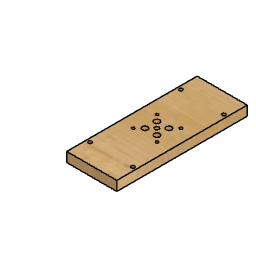
GaugePlate (Autodesk Fusion 360 design; units mm, degrees)
Autodesk Fusion 360 part; units mm, degrees
note: some values were not read from the file. Set by a fixed rule: which sketch regions a step uses.
sketch "Sketch1" plane through (-259.7942, 1290.9997, 156.4644) normal (0, 0, -1) x (0, -1, 0)
  arc A0 (507.289, -372.5213) -> (507.289, -319.0933) centre (371.7199, -345.8073) ccw
  arc A1 (507.289, -319.0933) -> (502.554, -315.2003) centre (502.554, -320.0263) ccw
  line L0 (502.554, -315.2003) -> (467.3804, -315.2003)
  arc A2 (467.3804, -315.2003) -> (465.9577, -315.4148) centre (467.3804, -320.0263) ccw
  arc A3 (452.8026, -315.6592) -> (465.9577, -315.4148) centre (458.9562, -292.7213) ccw
  arc A4 (452.8026, -315.6592) -> (450.3016, -315.6592) centre (451.5521, -320.3204) ccw
  arc A5 (437.9944, -315.6592) -> (450.3016, -315.6592) centre (444.148, -292.7213) ccw
  arc A6 (437.9944, -315.6592) -> (435.4934, -315.6592) centre (436.7439, -320.3204) ccw
  arc A7 (423.1862, -315.6592) -> (435.4934, -315.6592) centre (429.3398, -292.7213) ccw
  arc A8 (423.1862, -315.6592) -> (420.6852, -315.6592) centre (421.9357, -320.3204) ccw
  arc A9 (407.5301, -315.4148) -> (420.6852, -315.6592) centre (414.5316, -292.7213) ccw
  arc A10 (407.5301, -315.4148) -> (406.1074, -315.2003) centre (406.1074, -320.0263) ccw
  line L1 (406.1074, -315.2003) -> (370.9579, -315.2003)
  circle A11 centre (370.9579, -318.3753) radius 3.175
  line L2 (370.9579, -315.2003) -> (370.9338, -315.2003)
  arc A12 (370.9338, -315.2003) -> (366.1989, -319.0933) centre (370.9338, -320.0263) ccw
  arc A13 (366.1989, -319.0933) -> (366.1989, -372.5213) centre (501.7679, -345.8073) ccw
  arc A14 (366.1989, -372.5213) -> (370.9338, -376.4143) centre (370.9338, -371.5883) ccw
  line L3 (370.9338, -376.4143) -> (406.1074, -376.4143)
  arc A15 (406.1074, -376.4143) -> (407.5301, -376.1998) centre (406.1074, -371.5883) ccw
  arc A16 (420.6852, -375.9554) -> (407.5301, -376.1998) centre (414.5316, -398.8933) ccw
  arc A17 (420.6852, -375.9554) -> (423.1862, -375.9554) centre (421.9357, -371.2942) ccw
  arc A18 (435.4934, -375.9554) -> (423.1862, -375.9554) centre (429.3398, -398.8933) ccw
  arc A19 (435.4934, -375.9554) -> (437.9944, -375.9554) centre (436.7439, -371.2942) ccw
  arc A20 (450.3016, -375.9554) -> (437.9944, -375.9554) centre (444.148, -398.8933) ccw
  arc A21 (450.3016, -375.9554) -> (452.8026, -375.9554) centre (451.5521, -371.2942) ccw
  arc A22 (465.9577, -376.1998) -> (452.8026, -375.9554) centre (458.9562, -398.8933) ccw
  arc A23 (465.9577, -376.1998) -> (467.3804, -376.4143) centre (467.3804, -371.5883) ccw
  line L4 (467.3804, -376.4143) -> (502.5299, -376.4143)
  circle A24 centre (502.5299, -373.2393) radius 3.175
  line L5 (502.5299, -376.4143) -> (502.554, -376.4143)
  arc A25 (502.554, -376.4143) -> (507.289, -372.5213) centre (502.554, -371.5883) ccw
  circle A26 centre (500.2312, -363.2317) radius 0.8455
  circle A27 centre (472.3166, -363.2317) radius 0.8455
  circle A28 centre (379.5939, -318.8198) radius 2.159
  circle A29 centre (379.5939, -372.7948) radius 2.159
  circle A30 centre (478.3364, -363.2317) radius 2.159
  circle A31 centre (494.2114, -363.2317) radius 2.159
  circle A32 centre (493.8939, -372.7948) radius 2.159
  circle A33 centre (493.8939, -318.8198) radius 2.159
  circle A34 centre (436.7439, -345.8073) radius 6.35
  arc A35 (376.4189, -329.4243) -> (372.7359, -333.1073) centre (376.4189, -333.1073) ccw
  line L6 (376.4189, -329.4243) -> (382.7689, -329.4243)
  arc A36 (386.4519, -333.1073) -> (382.7689, -329.4243) centre (382.7689, -333.1073) ccw
  line L7 (386.4519, -333.1073) -> (386.4519, -358.5073)
  arc A37 (382.7689, -362.1903) -> (386.4519, -358.5073) centre (382.7689, -358.5073) ccw
  line L8 (382.7689, -362.1903) -> (376.4189, -362.1903)
  arc A38 (372.7359, -358.5073) -> (376.4189, -362.1903) centre (376.4189, -358.5073) ccw
  line L9 (372.7359, -358.5073) -> (372.7359, -333.1073)
  circle A39 centre (371.7439, -373.3073) radius 2.413
  circle A40 centre (501.7439, -318.3073) radius 2.413
  line L10 (518.7439, -314.3073) -> (354.7439, -314.3073)
  line L11 (354.7439, -314.3073) -> (354.7439, -377.3073)
  line L12 (354.7439, -377.3073) -> (518.7439, -377.3073)
  line L13 (518.7439, -377.3073) -> (518.7439, -314.3073)
  circle A41 centre (493.8939, -318.8198) radius 2.159
  circle A42 centre (493.8939, -372.7948) radius 2.159
  circle A43 centre (379.5939, -318.8198) radius 2.159
  circle A44 centre (379.5939, -372.7948) radius 2.159
  circle A45 centre (436.7439, -345.8073) radius 2.3876
  dimension "GaugePlateLength" = 164
  dimension "GaugePlateWidth" = 63
  dimension "d106" = 82
  dimension "d107" = 31.5
  constraint horizontal L10
  constraint vertical L11
  constraint horizontal L12
  constraint vertical L13
  constraint concentric A33 A41
  constraint concentric A32 A42
  constraint concentric A28 A43
  constraint concentric A29 A44
  measures "GaugePlateLength" distance of L10.start L10.end
  measures "GaugePlateWidth" distance of L10.start L12.end
  measures "d106" distance of A34.centre L13
  measures "d107" distance of A34.centre L10
extrude "Extrude1" add sketch "Sketch1" along normal blind 12.1 contours A0 A1 L0 A2 A3 A4 A5 A6 A7 A8 A9 A10 L1 A11 A12 A13 A14 L3 A15 A16 A17 A18 A19 A20 A21 A22 A23 L4 A24 A25 | A24 L5 | A11 L2 | A26 | A27 | A30 | A31 | A34 | A35 L6 A36 L7 A37 L8 A38 L9 | A39 | A40 | L10 L11 L12 L13
move_body "Move1" bodies 1 to x (1, 0, 0) y (0, 1, 0) z (0, 0, 1) at (0, -10, 0)
sketch "Sketch2" plane through (0, 0, 156.4644) normal (0, 0, 1) x (-1, 0, 0)
  circle A0 centre (-493.8939, -308.8198) radius 2.159
  circle A1 centre (-493.8939, -362.7948) radius 2.159
  circle A2 centre (-379.5939, -362.7948) radius 2.159
  circle A3 centre (-379.5939, -308.8198) radius 2.159
  line L0 (-518.7439, -304.3073) -> (-518.7439, -367.3073)
  line L1 (-518.7439, -367.3073) -> (-354.7439, -367.3073)
  line L2 (-354.7439, -367.3073) -> (-354.7439, -304.3073)
  line L3 (-354.7439, -304.3073) -> (-518.7439, -304.3073)
  circle A4 centre (-616.7439, -343.8073) radius 1.75
  circle A5 centre (-646.7439, -343.8073) radius 1.75
  circle A6 centre (-616.7439, -313.8073) radius 1.75
  circle A7 centre (-646.7439, -313.8073) radius 1.75
  circle A8 centre (-436.7439, -335.8073) radius 2.3876
sketch "Sketch3" plane through (0, 0, 156.4644) normal (0, 0, 1) x (-1, 0, 0)
  circle A0 centre (-59.0256, -787.1058) radius 2.159
  circle A1 centre (-113.0006, -787.1058) radius 2.159
  circle A2 centre (-113.0006, -901.4058) radius 2.159
  circle A3 centre (-59.0256, -901.4058) radius 2.159
  line L0 (-54.5131, -762.2558) -> (-117.5131, -762.2558)
  line L1 (-117.5131, -762.2558) -> (-117.5131, -926.2558)
  line L2 (-117.5131, -926.2558) -> (-54.5131, -926.2558)
  line L3 (-54.5131, -926.2558) -> (-54.5131, -762.2558)
  circle A4 centre (-71.0131, -859.2558) radius 1.75
  circle A5 centre (-101.0131, -859.2558) radius 1.75
  circle A6 centre (-71.0131, -829.2558) radius 1.75
  circle A7 centre (-101.0131, -829.2558) radius 1.75
  circle A8 centre (-78.5131, -851.7558) radius 3.5
  circle A9 centre (-86.0131, -844.2558) radius 2.3876
  circle A10 centre (-86.0131, -844.2558) radius 2.6126
  circle A11 centre (-93.5131, -851.7558) radius 3.5
  circle A12 centre (-78.5131, -836.7558) radius 3.5
  circle A13 centre (-93.5131, -836.7558) radius 3.5
  dimension "d120" = 3.5
  dimension "d124" = 30
  dimension "d166" = 7
  dimension "d169" = 15
  dimension "d170" = 15
  dimension "d171" = 7.5
  dimension "d172" = 7.5
  dimension "d173" = 0.225
  dimension "d176" = -15
  dimension "d177" = 15
  measures "d120" diameter of A4
  measures "d166" diameter of A8
  measures "d169" horizontal distance of A4.centre A9.centre
  measures "d170" vertical distance of A4.centre A9.centre
  measures "d171" horizontal distance of A8.centre A9.centre
  measures "d172" vertical distance of A8.centre A9.centre
extrude "Extrude3" cut sketch "Sketch3" against normal blind 12.3 contours A4 | A5 | A6 | A7 | A8 | A10 | A11 | A12 | A13
equation "d106 = GaugePlateLength / 2"
equation "d107 = GaugePlateWidth / 2"
equation "GaugePlateHeight = 12.1 mm"
equation "d120 = CarriageScrewDiameter"
equation "d123 = -CarriageScrewSeparation"
equation "d124 = CarriageScrewSeparation"
equation "CarriageScrewDiameter = 3.5 mm"
equation "CarriageScrewSeparation = 30.00 mm"
